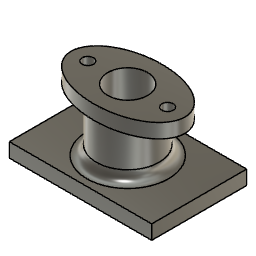
Stuffing_Box_Assembly (Autodesk Fusion 360 archive; units mm, degrees)
design "body 1"
Autodesk Fusion 360 part; units mm, degrees
note: some values were not read from the file. Set by a fixed rule: which face or edge a step refers to.
sketch "Sketch1" plane through (0, 0, 0) normal (0, 1, 0) x (1, 0, 0)
  line L0 (-0.298, 24.9818) -> (-0.298, 39.9818)
  line L1 (20.702, -25.0182) -> (20.702, 21.9818)
  line L2 (32.702, -25.0182) -> (20.702, -25.0182)
  line L3 (-0.298, 24.9818) -> (-0.298, 39.9818)
  line L4 (-0.298, 39.9818) -> (-0.298, 24.9818)
  line L5 (20.702, -25.0182) -> (32.702, -25.0182)
  line L6 (32.702, -25.0182) -> (32.702, 14.9818)
  line L7 (32.702, 24.9818) -> (20.702, 24.9818)
  arc A0 (42.702, 24.9818) -> (32.702, 14.9818) centre (42.702, 14.9818) ccw
  line L8 (20.702, 24.9818) -> (42.702, 24.9818)
  line L9 (-0.298, 24.9818) -> (-0.298, -40.0182)
  line L10 (20.702, 20.4995) -> (20.702, 24.9818)
  dimension "d3" = 15
  dimension "d10" = 15
  dimension "d13" = 10
  constraint vertical L0
  constraint vertical L1
  constraint horizontal L2
  constraint vertical L4
  constraint horizontal L5
  constraint vertical L6
  constraint horizontal L7
  constraint coincident L7.start L6
  constraint tangent L6 A0
  constraint tangent A0 L8
  constraint vertical L10
  constraint coincident L1 L10.start
  measures "d3" distance of L0.end L0.start
  measures "d10" distance of L0.start L0.end
  measures "d13" radius of A0
revolve "Revolve1" add sketch "Sketch1" angle 360 about axis through (-0.298, 0, -24.9818) along (0, 0, 1)
sketch "Sketch2" plane through (0, 0, 25.0182) normal (0, 0, 1) x (-1, 0, 0)
  circle A0 centre (0.298, 0) radius 33
  circle A1 centre (0.298, 0) radius 21
  ellipse E0 centre (0, 0) end of major axis (60, 0) minor radius 36
  line L0 (-60, 0) -> (60, 0)
  line L1 (0, -36) -> (0, 36)
  dimension "d15" = 120
  dimension "d16" = 72
  constraint coincident E0 L0.start
  constraint coincident E0 L0.end
  constraint coincident E0 L1.start
  constraint coincident E0 L1.end
  constraint coincident E0.centre origin
  constraint horizontal L0
  measures "d15" distance of E0
extrude "Extrude1" add sketch "Sketch2" along normal blind 15 contours A0 A1 L0 L1 | A0 E0 L0 L1 | A0 A1 L0 L1 | A0 E0 L0 L1 | A0 A1 L0 L1 | A0 E0 L0 L1 | A0 E0 L0 L1 | A0 A1 L0 L1
sketch "Sketch3" plane through (0, 0, -24.9818) normal (0, 0, -1) x (1, 0, 0)
  circle A0 centre (-0.298, 0) radius 21
  circle A1 centre (-0.298, 0) radius 43
  line L0 (75, -50) -> (-75, -50)
  line L1 (-75, -50) -> (-75, 50)
  line L2 (-75, 50) -> (75, 50)
  line L3 (75, 50) -> (75, -50)
  circle A2 centre (-0.298, 0) radius 16.5
  dimension "d19" = 33
  constraint horizontal L0
  constraint vertical L1
  constraint horizontal L2
  constraint vertical L3
  constraint concentric A0 A2
  measures "d19" diameter of A2
extrude "Extrude2" add sketch "Sketch3" along normal blind 15 contours A0 | A1 | L0 L1 L2 L3
fillet "Fillet1" radius 3 1 edges at (-31.0648, -11.9333, 25.0182)
sketch "Sketch4" plane through (0, 0, 40.0182) normal (0, 0, 1) x (-1, 0, 0)
  circle A0 centre (0.298, 0) radius 21
  ellipse E0 centre (0, 0) end of major axis (60, 0) minor radius 36
  circle A1 centre (42.298, 0) radius 6
  circle A2 centre (-41.702, 0) radius 6
  dimension "d24" = 42
  dimension "d25" = 84
  dimension "d26" = 12
  dimension "d27" = 12
  measures "d24" distance of A0.centre A2.centre
  measures "d25" distance of A1.centre A2.centre
  measures "d26" diameter of A1
  measures "d27" diameter of A2
extrude "Extrude3" cut sketch "Sketch4" against normal blind 35 contours A1 | A2

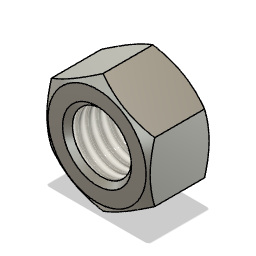
design "Hexagon Regular Nut ISO 4032 - M12 Steel 6 Plain"
description: Hexagon Regular Nut ISO 4032 - M12
part number: 2
Autodesk Fusion 360 part; units mm, degrees
sketch "Sketch1" plane through (0, 0, 0) normal (0, 1, 0) x (1, 0, 0)
  line L0 (0, 0.8114) -> (0, -2.1886)
  line L1 (-6, 0) -> (-8.55, 0)
  line L2 (-8.55, 0) -> (-10.395, -1.0652)
  line L3 (-10.395, -1.0652) -> (-10.395, -9.7348)
  line L4 (-10.395, -9.7348) -> (-8.55, -10.8)
  line L5 (-8.55, -10.8) -> (-6, -10.8)
  line L6 (-6, -10.8) -> (-6, 0)
  dimension "d121" = 12
  dimension "d122" = 30
  dimension "d123" = 30
  dimension "d125" = 17.1
  dimension "d126" = 10.8
  dimension "d127" = 17.1
  dimension "d128" = 20.79
  constraint vertical L0
  constraint coincident L0 L0.end
  constraint coincident origin L0
  constraint horizontal L1
  constraint perpendicular L1 L3
  constraint perpendicular L3 L5
  constraint perpendicular L5 L6
  constraint coincident origin L1
  measures "d122" angle of L1 L2
  measures "d123" angle of L4 L5
  measures "d126" distance of L1.start L5.end
revolve "Revolve1" add sketch "Sketch1" angle 360 about axis through (0, 0, -0.8114) along (0, 0, 1)
sketch "Sketch8" plane through (0, 0, 10.8) normal (0, 0, 1) x (1, 0, 0)
  line L0 (0, 0) -> (-18, 0) construction
  line L1 (-9, -5.2015) -> (-9, 5.2015)
  circle A0 centre (0, 0) radius 6
  circle A1 centre (0, 0) radius 10.395
  dimension "d114" = 9
  constraint horizontal L0
  constraint perpendicular L0 L1
  constraint midpoint L0 L1
  constraint coincident L0.start A0.centre
  constraint coincident L1.end A1
  measures "d114" distance of L0.start L1
extrude "Extrude5" cut sketch "Sketch8" against normal blind 10.8 contours L1 A1 picked at (-9.2251, -1.2669)
pattern_circular "C-Pattern2" count 6 over 360 about axis through (0, 0, 1.75) along (0, 0, 1) of "Extrude5"
thread "Thread3" "ISO Metric profile 12.0 M12x1.75 6H" major diameter 12.2265 minor diameter 10.2735 pitch 1.75 angle 60 resizes the face on face at (-5.9925, 0.2991, 7.2)
sketch "Sketch12" plane through (0, 0, 0) normal (0, 1, 0) x (1, 0, 0)
  line L0 (5.1368, -10.8) -> (-5.1368, -10.8)
  line L1 (8.55, -10.8) -> (-8.55, -10.8)
  line L2 (8.55, 0) -> (-8.55, 0)
  line L3 (5.1368, 0) -> (-5.1368, 0)
  line L4 (-6, 0) -> (-4.2, 0)
  line L5 (-4.2, 0) -> (-4.2, -1.8)
  line L6 (-4.2, -1.8) -> (-6, 0)
  line L7 (-6, -10.8) -> (-4.2, -10.8)
  line L8 (-4.2, -10.8) -> (-4.2, -9)
  line L9 (-4.2, -9) -> (-6, -10.8)
  line L10 (0, -1.75) -> (0, -22.5)
  dimension "d165" = 45
  dimension "d166" = 6
  dimension "d167" = 1.8
  dimension "d169" = 45
  constraint horizontal L4
  constraint perpendicular L4 L5
  constraint perpendicular L5 L7
  constraint perpendicular L2 L8
  constraint equal L5 L8
  constraint collinear L1 L7
  constraint collinear L2 L4
  constraint collinear L5 L8
  measures "d165" angle of L2 L6
  measures "d166" distance of L4.start L10
  measures "d167" distance of L4.end L5.end
  measures "d169" angle of L7 L9
revolve "Revolve3" cut sketch "Sketch12" angle 360 about axis through (0, 0, 1.75) along (0, 0, 1)
equation "adsk_nheig = 10.80 mm"
equation "adsk_maxdia = 20.79 mm"
equation "adsk_nomdia = 12.00 mm"
equation "d89 = -adsk_nheig"
equation "adsk_waflat = 18.00 mm"
equation "d114 = adsk_waflat / 2"
equation "adsk_chamang1 = 30.00 deg"
equation "adsk_chamang2 = 30.00 deg"
equation "d121 = adsk_nomdia"
equation "d122 = adsk_chamang1"
equation "d123 = adsk_chamang2"
equation "d125 = adsk_waflat * 0.95"
equation "d126 = adsk_nheig"
equation "d127 = adsk_waflat * 0.95"
equation "d128 = adsk_maxdia"
equation "d163 = adsk_nheig"
equation "d166 = adsk_nomdia * 0.5"
equation "d167 = adsk_nomdia * 0.15"

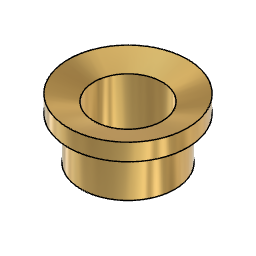
design "bush"
Autodesk Fusion 360 part; units mm, degrees
sketch "Sketch1" plane through (0, 0, 0) normal (0, 1, 0) x (1, 0, 0)
  line L0 (0, 10) -> (0, -11)
  line L1 (12, 10) -> (16.5, 10)
  line L2 (16.5, 10) -> (16.5, -5)
  line L3 (21, -11) -> (21, -5)
  line L4 (21, -5) -> (16.5, -5)
  line L5 (12, 10) -> (12, -8.5885)
  line L6 (21, -11) -> (12, -8.5885)
  dimension "d1" = 21
  dimension "d3" = 16.5
  dimension "d4" = 15
  dimension "d5" = 21
  dimension "d6" = 12
  constraint vertical L0
  constraint perpendicular L0 L1
  constraint perpendicular L1 L2
  constraint perpendicular L2 L4
  measures "d1" distance of L0.start L0.end
  measures "d3" distance of L0.start L1.end
  measures "d4" distance of L1.end L2.end
  measures "d5" distance of L0.end L3.start
  measures "d6" distance of L0.start L1.start
revolve "Revolve1" add sketch "Sketch1" angle 360 about axis through (0, 0, -10) along (0, 0, 1)

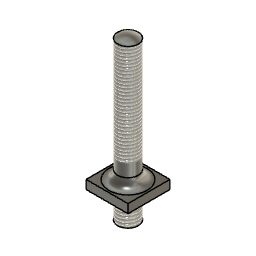
design "stud"
Autodesk Fusion 360 part; units mm, degrees
sketch "Sketch1" plane through (0, 0, 0) normal (0, 1, 0) x (1, 0, 0)
sketch "Sketch2" plane through (0, 0, 0) normal (0, 1, 0) x (1, 0, 0)
sketch "Sketch3" plane through (0, 0, 0) normal (0, 1, 0) x (1, 0, 0)
  line L0 (200, -50) -> (200, 40)
  line L1 (200, 40) -> (200, 25)
  line L2 (206, 25) -> (224, 25)
  line L3 (224, 25) -> (224, 20)
  line L4 (200, 20) -> (200, 25)
  line L5 (212, 25) -> (206, 25)
  line L6 (200, 25) -> (200, 40)
  line L7 (200, 8) -> (200, -50)
  line L8 (214.0559, 20) -> (213.2934, 20)
  line L9 (200, 20) -> (200, 8)
  line L10 (214.0559, 20) -> (224, 20)
  line L11 (206, -50) -> (206, 8)
  line L12 (200, 8) -> (200, -50)
  line L13 (200, 20) -> (200, 8)
  line L14 (206, 25) -> (206, 40)
  line L15 (200, 40) -> (200, 25)
  line L16 (200, -50) -> (200, -52)
  arc A0 (200, -52) -> (206, -50) centre (199.8414, -41.5243) ccw
  line L17 (213.2934, 20) -> (208.2934, 20)
  line L18 (200, 40) -> (200, 41)
  arc A1 (206, 40) -> (200, 41) centre (199.8072, 21.3429) ccw
  line L19 (206, 8) -> (206, 20)
  line L20 (206, 20) -> (208.2934, 20)
  dimension "d6" = 90
  dimension "d7" = 15
  dimension "d8" = 24
  dimension "d10" = 58
  dimension "d12" = 6
  dimension "d13" = 6
  dimension "d14" = 15
  constraint vertical L0
  constraint parallel L0 L1
  constraint horizontal L2
  constraint vertical L3
  constraint vertical L4
  constraint horizontal L5
  constraint vertical L6
  constraint vertical L7
  constraint horizontal L8
  constraint vertical L9
  constraint perpendicular L3 L10
  constraint vertical L11
  constraint vertical L12
  constraint vertical L13
  constraint vertical L14
  constraint vertical L15
  constraint coincident L4.start L8
  constraint coincident L2 L5.start
  constraint perpendicular L17 L19
  measures "d6" distance of L0.start L0.end
  measures "d7" distance of L0.end L1.end
  measures "d8" distance of L1.end L2.end
  measures "d10" distance of L0.start L7.start
  measures "d12" distance of L0.start L11.start
  measures "d13" distance of L1.end L2.start
  measures "d14" distance of L1.end L0.end
revolve "Revolve1" add sketch "Sketch3" angle 360 about axis through (200, 0, -8) along (0, 0, 1)
sketch "Sketch4" plane through (0, 0, -20) normal (0, 0, 1) x (-1, 0, 0)
  circle A0 centre (-200, 0) radius 24
  circle A1 centre (-200, 0) radius 6
  line L0 (-200, 0) -> (-200, 12)
  line L1 (-200, 12) -> (-212, 12)
  line L2 (-212, 12) -> (-188, 12)
  line L3 (-188, 12) -> (-188, -12)
  line L4 (-188, -12) -> (-212, -12)
  line L5 (-212, -12) -> (-212, 12)
  circle A2 centre (-200, 0) radius 24
  dimension "d17" = 12
  dimension "d18" = 12
  dimension "d19" = 24
  dimension "d20" = 24
  constraint coincident A0.centre A1.centre
  constraint vertical L0
  constraint perpendicular L0 L1
  constraint horizontal L2
  constraint vertical L3
  constraint horizontal L4
  constraint vertical L5
  measures "d17" distance of A0.centre L0.end
  measures "d18" distance of L0.end L1.end
  measures "d19" distance of L1.end L2.end
  measures "d20" distance of L1.end L4.end
extrude "Extrude1" cut sketch "Sketch4" against normal blind 100 contours A0 A2
fillet "Fillet1" radius 5 1 edges at (194.406, -2.1697, -20)
thread "Thread1" "ISO Metric profile 12.0 M12x1.75 6g" major diameter 11.8335 minor diameter 9.8365 pitch 1.75 angle 60 resizes the face on face at (197.2627, -5.3392, 28.3333) from (200, 0, -8) to (200, 0, 50)
thread "Thread2" "ISO Metric profile 12.0 M12x1.75 6g" major diameter 11.8335 minor diameter 9.8365 pitch 1.75 angle 60 resizes the face on face at (204.0788, -4.4004, -30)

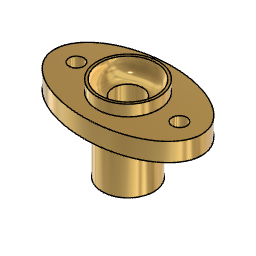
design "gland"
Autodesk Fusion 360 part; units mm, degrees
sketch "Sketch1" plane through (0, 0, 0) normal (0, 1, 0) x (1, 0, 0)
sketch "Sketch2" plane through (0, 0, 0) normal (0, 1, 0) x (1, 0, 0)
  line L0 (21, 0) -> (21, -45)
  line L1 (23, -69) -> (25, -69)
  line L2 (25, -69) -> (25, -60)
  line L3 (21, 0) -> (11.5798, -3.7681)
  line L4 (11.9227, -57) -> (11.5798, -3.7681)
  arc A0 (23, -69) -> (11, -57) centre (11, -69) ccw
  line L5 (0, 0) -> (0, -69)
  line L6 (0, -69) -> (0, -60)
  line L7 (11.9227, -57) -> (11.9229, -57.0355)
  line L8 (25, -60) -> (60, -60)
  line L9 (60, -60) -> (60, -45)
  line L10 (0, -45) -> (0, -60)
  line L11 (60, -45) -> (21, -45)
  dimension "d12" = 21
  dimension "d20" = 12
  dimension "d21" = 9
  dimension "d22" = 60
  dimension "d23" = 15
  constraint coincident L5.start origin
  constraint parallel L0 L5
  constraint parallel L5 L6
  constraint parallel L4 L7
  constraint coincident A0 L7.end
  constraint horizontal L8
  constraint vertical L9
  constraint horizontal L11
  constraint vertical L10
  measures "d12" distance of L5.start L0.start
  measures "d20" radius of A0
  measures "d21" distance of L5.end L6.end
  measures "d22" distance of L6.end L8.end
  measures "d23" distance of L6.end L10.start
revolve "Revolve1" add sketch "Sketch2" angle 360 about axis through (0, 0, 45) along (0, 0, 1)
sketch "Sketch3" plane through (0, 0, 60) normal (0, 0, 1) x (-1, 0, 0)
  circle A0 centre (0, 0) radius 60
  circle A1 centre (0, 0) radius 25
  circle A2 centre (0, 0) radius 60
  ellipse E0 centre (0, 0) end of major axis (-60, 0) minor radius 36
  line L0 (60, 0) -> (-60, 0)
  line L1 (0, 36) -> (0, -36)
  dimension "d25" = 72
  constraint concentric A0 A2
  constraint coincident E0 L0.start
  constraint coincident E0 L0.end
  constraint coincident E0 L1.start
  constraint coincident E0 L1.end
  constraint concentric A2 E0
  constraint horizontal L0
extrude "Extrude1" cut sketch "Sketch3" against normal blind 15 contours A0 A2 E0 | A0 A2 E0
sketch "Sketch4" plane through (0, 0, 0) normal (0, 1, 0) x (1, 0, 0)
sketch "Sketch5" plane through (0, 0, 60) normal (0, 0, 1) x (-1, 0, 0)
  ellipse E0 centre (0, 0) end of major axis (-60, 0) minor radius 36
  circle A0 centre (0, 0) radius 25
  circle A1 centre (42, 0) radius 6
  circle A2 centre (-42, 0) radius 6
  dimension "d32" = 42
  dimension "d33" = 84
  dimension "d34" = 12
  dimension "d35" = 12
  measures "d32" distance of E0.centre A2.centre
  measures "d33" distance of A1.centre A2.centre
  measures "d34" diameter of A1
  measures "d35" diameter of A2
extrude "Extrude2" cut sketch "Sketch5" against normal blind 100 contours A1 | A2
